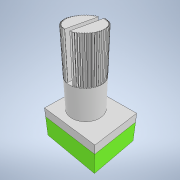
# Autodesk Inventor part: Потенциометр маленький
Saved by Autodesk Inventor 2021.1 (Build 251245010, 245A)
## iProperties
Created: 2022-06-30
Part Number: Потенциометр маленький
Material: Типовые
Document SubType Name: Modeling
Designer: Andrew
Density: 1 g/cm^3
Appearance: По умолчанию
Author: Andrew
Autodesk Inventor part; units mm, degrees
ref_plane "YZ Plane" through (0, 0, 0) normal (1, 0, 0) x (0, 1, 0)
ref_plane "XZ Plane" through (0, 0, 0) normal (0, 1, 0) x (-1, 0, 0)
ref_plane "XY Plane" through (0, 0, 0) normal (0, 0, 1) x (1, 0, 0)
sketch "Эскиз1" plane through (0, 0, 0) normal (0, 1, 0) x (-1, 0, 0)
  line L0 (7, 10) -> (-5, 10)
  line L1 (-5, 10) -> (-5, 0)
  line L2 (-5, 0) -> (7, 0)
  line L3 (7, 0) -> (7, 10)
  point P0 (0, 0)
  dimension "d0" = 12
  dimension "d1" = 10
  constraints: 8 end point, 2 parallel, 1 horizontal, 1 perpendicular
  measures "d0" distance of L2.end L1.end
  measures "d1" distance of L1.end L0.end
extrude "Выдавливание1" add sketch "Эскиз1" along normal blind 4.5
sketch "Эскиз2" plane through (0, 4.5, 0) normal (0, 1, 0) x (1, 0, 0)
  line L0 (-7, 0) -> (-7, -10) projected
  line L1 (5, -10) -> (5, 0) projected
  line L2 (-7, -10) -> (5, -10)
  line L3 (5, -10) -> (5, 0)
  line L4 (5, 0) -> (-7, 0)
  line L5 (-7, 0) -> (-7, -10)
  point P0 (0, 0)
  constraints: 8 end point, 2 parallel, 1 horizontal, 1 perpendicular
extrude "Выдавливание2" add sketch "Эскиз2" along normal blind 2 separate body
sketch "Эскиз3" plane through (0, 6.5, 0) normal (0, 1, 0) x (1, 0, 0)
  circle A0 centre (-2, -5) radius 3.5
  line L0 (5, 0) -> (-7, 0) projected
  line L1 (-7, 0) -> (-7, -10) projected
  point P0 (0, 0)
  dimension "d6" = 7
  dimension "d7" = 5
  dimension "d8" = 5
  constraints: 1 centre point
  measures "d6" diameter of A0
  measures "d7" distance from line of L0 A0.centre
  measures "d8" distance from line of L1 A0.centre
extrude "Выдавливание3" add sketch "Эскиз3" along normal blind 15 separate body
sketch "Эскиз4" plane through (-2, 21.5, 5) normal (0, 1, 0) x (1, 0, 0)
  circle A0 centre (0, 0) radius 3.5
  line L0 (-0.5, -3.4641) -> (-0.5, 3.4641)
  line L1 (0.5, -3.4641) -> (0.5, 3.4641)
  circle A1 centre (0, 0) radius 3.25
  line L2 (1.1998, -3.0204) -> (1.4364, -3.1917)
  line L3 (1.4364, -2.9153) -> (1.4364, -3.1917)
  line L4 (1.509, -2.8785) -> (1.7622, -3.024)
  line L5 (1.7333, -2.7492) -> (1.7622, -3.024)
  line L6 (1.8016, -2.705) -> (2.0686, -2.8233)
  line L7 (2.0112, -2.553) -> (2.0686, -2.8233)
  line L8 (2.0745, -2.5018) -> (2.3524, -2.5916)
  line L9 (2.267, -2.3288) -> (2.3524, -2.5916)
  line L10 (2.3246, -2.2713) -> (2.6104, -2.3315)
  line L11 (2.498, -2.079) -> (2.6104, -2.3315)
  line L12 (2.5493, -2.0158) -> (2.8398, -2.0458)
  line L13 (2.7017, -1.8065) -> (2.8398, -2.0458)
  line L14 (2.746, -1.7383) -> (3.0381, -1.7378)
  line L15 (2.8757, -1.5142) -> (3.0381, -1.7378)
  line L16 (2.9127, -1.4418) -> (3.2031, -1.4107)
  line L17 (3.0182, -1.2054) -> (3.2031, -1.4107)
  line L18 (3.0474, -1.1294) -> (3.333, -1.0682)
  line L19 (3.1277, -0.8833) -> (3.333, -1.0682)
  line L20 (3.1488, -0.8047) -> (3.4264, -0.7139)
  line L21 (3.2029, -0.5515) -> (3.4264, -0.7139)
  line L22 (3.2157, -0.4711) -> (3.4823, -0.3518)
  line L23 (3.243, -0.2137) -> (3.4823, -0.3518)
  line L24 (3.2473, -0.1324) -> (3.5, 0.0141)
  line L25 (3.2475, 0.1265) -> (3.5, 0.0141)
  line L26 (3.2434, 0.2077) -> (3.4793, 0.3799)
  line L27 (3.2165, 0.4652) -> (3.4793, 0.3799)
  line L28 (3.2039, 0.5456) -> (3.4206, 0.7415)
  line L29 (3.1503, 0.7989) -> (3.4206, 0.7415)
  line L30 (3.1293, 0.8775) -> (3.3243, 1.0949)
  line L31 (3.0495, 1.1238) -> (3.3243, 1.0949)
  line L32 (3.0204, 1.1998) -> (3.1917, 1.4364)
  line L33 (2.9153, 1.4364) -> (3.1917, 1.4364)
  line L34 (2.8785, 1.509) -> (3.024, 1.7622)
  line L35 (2.7492, 1.7333) -> (3.024, 1.7622)
  line L36 (2.705, 1.8016) -> (2.8233, 2.0686)
  line L37 (2.553, 2.0112) -> (2.8233, 2.0686)
  line L38 (2.5018, 2.0745) -> (2.5916, 2.3524)
  line L39 (2.3288, 2.267) -> (2.5916, 2.3524)
  line L40 (2.2713, 2.3246) -> (2.3315, 2.6104)
  line L41 (2.079, 2.498) -> (2.3315, 2.6104)
  line L42 (2.0158, 2.5493) -> (2.0458, 2.8398)
  line L43 (1.8065, 2.7017) -> (2.0458, 2.8398)
  line L44 (1.7383, 2.746) -> (1.7378, 3.0381)
  line L45 (1.5142, 2.8757) -> (1.7378, 3.0381)
  line L46 (1.4418, 2.9127) -> (1.4107, 3.2031)
  line L47 (1.2054, 3.0182) -> (1.4107, 3.2031)
  line L48 (1.1294, 3.0474) -> (1.0682, 3.333)
  line L49 (0.8833, 3.1277) -> (1.0682, 3.333)
  line L50 (0.8047, 3.1488) -> (0.7139, 3.4264)
  line L51 (0.5515, 3.2029) -> (0.7139, 3.4264)
  line L52 (0.4711, 3.2157) -> (0.3518, 3.4823)
  line L53 (0.2137, 3.243) -> (0.3518, 3.4823)
  line L54 (0.1324, 3.2473) -> (-0.0141, 3.5)
  line L55 (-0.1265, 3.2475) -> (-0.0141, 3.5)
  line L56 (-0.2077, 3.2434) -> (-0.3799, 3.4793)
  line L57 (-0.4652, 3.2165) -> (-0.3799, 3.4793)
  line L58 (-0.5456, 3.2039) -> (-0.7415, 3.4206)
  line L59 (-0.7989, 3.1503) -> (-0.7415, 3.4206)
  line L60 (-0.8775, 3.1293) -> (-1.0949, 3.3243)
  line L61 (-1.1238, 3.0495) -> (-1.0949, 3.3243)
  line L62 (-1.1998, 3.0204) -> (-1.4364, 3.1917)
  line L63 (-1.4364, 2.9153) -> (-1.4364, 3.1917)
  line L64 (-1.509, 2.8785) -> (-1.7622, 3.024)
  line L65 (-1.7333, 2.7492) -> (-1.7622, 3.024)
  line L66 (-1.8016, 2.705) -> (-2.0686, 2.8233)
  line L67 (-2.0112, 2.553) -> (-2.0686, 2.8233)
  line L68 (-2.0745, 2.5018) -> (-2.3524, 2.5916)
  line L69 (-2.267, 2.3288) -> (-2.3524, 2.5916)
  line L70 (-2.3246, 2.2713) -> (-2.6104, 2.3315)
  line L71 (-2.498, 2.079) -> (-2.6104, 2.3315)
  line L72 (-2.5493, 2.0158) -> (-2.8398, 2.0458)
  line L73 (-2.7017, 1.8065) -> (-2.8398, 2.0458)
  line L74 (-2.746, 1.7383) -> (-3.0381, 1.7378)
  line L75 (-2.8757, 1.5142) -> (-3.0381, 1.7378)
  line L76 (-2.9127, 1.4418) -> (-3.2031, 1.4107)
  line L77 (-3.0182, 1.2054) -> (-3.2031, 1.4107)
  line L78 (-3.0474, 1.1294) -> (-3.333, 1.0682)
  line L79 (-3.1277, 0.8833) -> (-3.333, 1.0682)
  line L80 (-3.1488, 0.8047) -> (-3.4264, 0.7139)
  line L81 (-3.2029, 0.5515) -> (-3.4264, 0.7139)
  line L82 (-3.2157, 0.4711) -> (-3.4823, 0.3518)
  line L83 (-3.243, 0.2137) -> (-3.4823, 0.3518)
  line L84 (-3.2473, 0.1324) -> (-3.5, -0.0141)
  line L85 (-3.2475, -0.1265) -> (-3.5, -0.0141)
  line L86 (-3.2434, -0.2077) -> (-3.4793, -0.3799)
  line L87 (-3.2165, -0.4652) -> (-3.4793, -0.3799)
  line L88 (-3.2039, -0.5456) -> (-3.4206, -0.7415)
  line L89 (-3.1503, -0.7989) -> (-3.4206, -0.7415)
  line L90 (-3.1293, -0.8775) -> (-3.3243, -1.0949)
  line L91 (-3.0495, -1.1238) -> (-3.3243, -1.0949)
  line L92 (-3.0204, -1.1998) -> (-3.1917, -1.4364)
  line L93 (-2.9153, -1.4364) -> (-3.1917, -1.4364)
  line L94 (-2.8785, -1.509) -> (-3.024, -1.7622)
  line L95 (-2.7492, -1.7333) -> (-3.024, -1.7622)
  line L96 (-2.705, -1.8016) -> (-2.8233, -2.0686)
  line L97 (-2.553, -2.0112) -> (-2.8233, -2.0686)
  line L98 (-2.5018, -2.0745) -> (-2.5916, -2.3524)
  line L99 (-2.3288, -2.267) -> (-2.5916, -2.3524)
  line L100 (-2.2713, -2.3246) -> (-2.3315, -2.6104)
  line L101 (-2.079, -2.498) -> (-2.3315, -2.6104)
  line L102 (-2.0158, -2.5493) -> (-2.0458, -2.8398)
  line L103 (-1.8065, -2.7017) -> (-2.0458, -2.8398)
  line L104 (-1.7383, -2.746) -> (-1.7378, -3.0381)
  line L105 (-1.5142, -2.8757) -> (-1.7378, -3.0381)
  line L106 (-1.4418, -2.9127) -> (-1.4107, -3.2031)
  line L107 (-1.2054, -3.0182) -> (-1.4107, -3.2031)
  line L108 (-1.1294, -3.0474) -> (-1.0682, -3.333)
  line L109 (-0.8833, -3.1277) -> (-1.0682, -3.333)
  line L110 (-0.8047, -3.1488) -> (-0.7139, -3.4264)
  line L111 (-0.5515, -3.2029) -> (-0.7139, -3.4264)
  line L112 (-0.4711, -3.2157) -> (-0.3518, -3.4823)
  line L113 (-0.2137, -3.243) -> (-0.3518, -3.4823)
  line L114 (-0.1324, -3.2473) -> (0.0141, -3.5)
  line L115 (0.1265, -3.2475) -> (0.0141, -3.5)
  line L116 (0.2077, -3.2434) -> (0.3799, -3.4793)
  line L117 (0.4652, -3.2165) -> (0.3799, -3.4793)
  line L118 (0.5456, -3.2039) -> (0.7415, -3.4206)
  line L119 (0.7989, -3.1503) -> (0.7415, -3.4206)
  line L120 (0.8775, -3.1293) -> (1.0949, -3.3243)
  line L121 (1.1238, -3.0495) -> (1.0949, -3.3243)
  point P0 (2, 5)
  point P1 (0.7415, -3.4206)
  point P2 (0.7415, -3.4206)
  point P3 (0.7415, -3.4206)
  point P4 (-0.7139, -3.4264)
  point P5 (-0.7139, -3.4264)
  point P6 (-0.7139, -3.4264)
  point P7 (-0.8047, -3.1488)
  point P8 (-1.0682, -3.333)
  point P9 (-1.0682, -3.333)
  point P10 (-1.0682, -3.333)
  point P11 (-1.1294, -3.0474)
  point P12 (-1.2054, -3.0182)
  point P13 (-1.4107, -3.2031)
  point P14 (-1.4107, -3.2031)
  point P15 (-1.4107, -3.2031)
  point P16 (-1.4418, -2.9127)
  point P17 (-1.5142, -2.8757)
  point P18 (-1.7378, -3.0381)
  point P19 (-1.7378, -3.0381)
  point P20 (-1.7378, -3.0381)
  point P21 (-1.7383, -2.746)
  point P22 (-1.8065, -2.7017)
  point P23 (-2.0458, -2.8398)
  point P24 (-2.0458, -2.8398)
  point P25 (-2.0458, -2.8398)
  point P26 (-2.0158, -2.5493)
  point P27 (-2.3315, -2.6104)
  point P28 (-2.3315, -2.6104)
  point P29 (-2.3315, -2.6104)
  point P30 (-2.2713, -2.3246)
  point P31 (-2.3288, -2.267)
  point P32 (-2.5916, -2.3524)
  point P33 (-2.5916, -2.3524)
  point P34 (-2.5916, -2.3524)
  point P35 (-2.5018, -2.0745)
  point P36 (-2.553, -2.0112)
  point P37 (-2.8233, -2.0686)
  point P38 (-2.8233, -2.0686)
  point P39 (-2.8233, -2.0686)
  point P40 (-2.705, -1.8016)
  point P41 (-2.7492, -1.7333)
  point P42 (-3.024, -1.7622)
  point P43 (-3.024, -1.7622)
  point P44 (-3.024, -1.7622)
  point P45 (-2.8785, -1.509)
  point P46 (-2.9153, -1.4364)
  point P47 (-3.1917, -1.4364)
  point P48 (-3.1917, -1.4364)
  point P49 (-3.1917, -1.4364)
  point P50 (-3.0204, -1.1998)
  point P51 (-3.0495, -1.1238)
  point P52 (-3.3243, -1.0949)
  point P53 (-3.3243, -1.0949)
  point P54 (-3.3243, -1.0949)
  point P55 (-3.1293, -0.8775)
  point P56 (-3.1503, -0.7989)
  point P57 (-3.4206, -0.7415)
  point P58 (-3.4206, -0.7415)
  point P59 (-3.4206, -0.7415)
  point P60 (-3.2039, -0.5456)
  point P61 (-3.2434, -0.2077)
  point P62 (-3.2475, -0.1265)
  point P63 (-3.2473, 0.1324)
  point P64 (-3.243, 0.2137)
  point P65 (-3.4823, 0.3518)
  point P66 (-3.4823, 0.3518)
  point P67 (-3.4823, 0.3518)
  point P68 (-3.2157, 0.4711)
  point P69 (-3.4264, 0.7139)
  point P70 (-3.4264, 0.7139)
  point P71 (-3.4264, 0.7139)
  point P72 (-3.1488, 0.8047)
  point P73 (-3.333, 1.0682)
  point P74 (-3.333, 1.0682)
  point P75 (-3.333, 1.0682)
  point P76 (-3.0474, 1.1294)
  point P77 (-3.0182, 1.2054)
  point P78 (-3.2031, 1.4107)
  point P79 (-3.2031, 1.4107)
  point P80 (-3.2031, 1.4107)
  point P81 (-2.7017, 1.8065)
  point P82 (-2.5493, 2.0158)
  point P83 (-2.6104, 2.3315)
  point P84 (-2.6104, 2.3315)
  point P85 (-2.6104, 2.3315)
  point P86 (-2.3246, 2.2713)
  point P87 (-2.267, 2.3288)
  point P88 (-1.7622, 3.024)
  point P89 (-1.7622, 3.024)
  point P90 (-1.7622, 3.024)
  point P91 (-1.1998, 3.0204)
  point P92 (-1.1238, 3.0495)
  point P93 (-1.0949, 3.3243)
  point P94 (-1.0949, 3.3243)
  point P95 (-1.0949, 3.3243)
  point P96 (-0.8775, 3.1293)
  point P97 (-0.7989, 3.1503)
  point P98 (-0.7415, 3.4206)
  point P99 (-0.7415, 3.4206)
  point P100 (-0.7415, 3.4206)
  point P101 (-0.5, 3.2113)
  point P102 (-0.5, -3.2113)
  point P103 (-0.5515, -3.2029)
  point P104 (0.5456, -3.2039)
  point P105 (0.5, -3.2113)
  point P106 (0.5, 3.2113)
  point P107 (2.5916, 2.3524)
  point P108 (2.5916, 2.3524)
  point P109 (2.5916, 2.3524)
  point P110 (2.7492, 1.7333)
  point P111 (3.024, 1.7622)
  point P112 (3.024, 1.7622)
  point P113 (3.024, 1.7622)
  point P114 (2.8785, 1.509)
  point P115 (3.0204, 1.1998)
  point P116 (3.0495, 1.1238)
  point P117 (3.1293, 0.8775)
  point P118 (3.4206, 0.7415)
  point P119 (3.4206, 0.7415)
  point P120 (3.4206, 0.7415)
  point P121 (3.2039, 0.5456)
  point P122 (3.2165, 0.4652)
  point P123 (3.4793, 0.3799)
  point P124 (3.4793, 0.3799)
  point P125 (3.4793, 0.3799)
  point P126 (3.2434, 0.2077)
  point P127 (3.5, 0.0141)
  point P128 (3.5, 0.0141)
  point P129 (3.5, 0.0141)
  point P130 (3.2473, -0.1324)
  point P131 (3.243, -0.2137)
  point P132 (3.4823, -0.3518)
  point P133 (3.4823, -0.3518)
  point P134 (3.4823, -0.3518)
  point P135 (3.2157, -0.4711)
  point P136 (3.2029, -0.5515)
  point P137 (3.4264, -0.7139)
  point P138 (3.4264, -0.7139)
  point P139 (3.4264, -0.7139)
  point P140 (3.1488, -0.8047)
  point P141 (3.1277, -0.8833)
  point P142 (3.333, -1.0682)
  point P143 (3.333, -1.0682)
  point P144 (3.333, -1.0682)
  point P145 (3.0474, -1.1294)
  point P146 (3.0182, -1.2054)
  point P147 (3.0381, -1.7378)
  point P148 (3.0381, -1.7378)
  point P149 (3.0381, -1.7378)
  point P150 (2.498, -2.079)
  point P151 (2.6104, -2.3315)
  point P152 (2.6104, -2.3315)
  point P153 (2.6104, -2.3315)
  point P154 (2.3246, -2.2713)
  point P155 (1.4364, -3.1917)
  point P156 (1.4364, -3.1917)
  point P157 (1.4364, -3.1917)
  dimension "d11" = 7
  dimension "d14" = 6.5
  dimension "d17" = 360
  constraints: 244 end point, 1 coincident, 369 other
extrude "Выдавливание4" cut sketch "Эскиз4" against normal blind 8.5 contours A0 L23 A1 L24 | L25 A1 L26 A0 | A0 L21 A1 L22 | L27 A1 L28 A0 | A0 L19 A1 L20 | L29 A1 L30 A0 | A0 L17 A1 L18 | L31 A1 L32 A0 | A0 L15 A1 L16 | L33 A1 L34 A0 | A0 L13 A1 L14 | L35 A1 L36 A0 | A0 L11 A1 L12 | L37 A1 L38 A0 | A0 L9 A1 L10 | L39 A1 L40 A0 | A0 L7 A1 L8 | L41 A1 L42 A0 | A0 L5 A1 L6 | L43 A1 L44 A0 | A0 L3 A1 L4 | L45 A1 L46 A0 | A0 L121 A1 L2 | L47 A1 L48 A0 | A0 L119 A1 L120 | L49 A1 L50 A0 | A0 L1 A1 L118 | L51 A1 L1 A0 | A0 L117 A1 L1 | L1 A1 L52 A0 | A0 L115 A1 L116 | L116 A1 L117 | A1 L0 L1 | L53 A1 L54 A0 | L52 A1 L53 | A0 L113 A1 L114 | L114 A1 L115 | L55 A1 L56 A0 | L54 A1 L55 | A0 L0 A1 L112 | L112 A1 L113 | L57 A1 L0 A0 | L56 A1 L57 | A0 L111 A1 L0 | L0 A1 L58 A0 | A0 L109 A1 L110 | L59 A1 L60 A0 | A0 L107 A1 L108 | L61 A1 L62 A0 | A0 L105 A1 L106 | L63 A1 L64 A0 | A0 L103 A1 L104 | L65 A1 L66 A0 | A0 L101 A1 L102 | L67 A1 L68 A0 | A0 L99 A1 L100 | L69 A1 L70 A0 | A0 L97 A1 L98 | L71 A1 L72 A0 | A0 L95 A1 L96 | L73 A1 L74 A0 | A0 L93 A1 L94 | L75 A1 L76 A0 | A0 L91 A1 L92 | L77 A1 L78 A0 | A0 L89 A1 L90 | L79 A1 L80 A0 | A0 L87 A1 L88 | L81 A1 L82 A0 | A0 L85 A1 L86 | L83 A1 L84 A0 bodies 3
